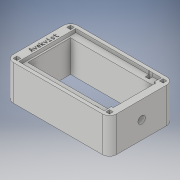
# Autodesk Inventor part: AttendMiddle
Saved by Autodesk Inventor 2019 (Build 230136000, 136)
## iProperties
Created: 2018-11-13
Part Number: AttendMiddle
Material: Generic
Document SubType Name: Modeling
Designer: hampu
Density: 1 g/cm^3
Appearance: Default
Author: hampu
Autodesk Inventor part; units mm, degrees
ref_plane "YZ Plane" through (0, 0, 0) normal (1, 0, 0) x (0, 1, 0)
ref_plane "XZ Plane" through (0, 0, 0) normal (0, 1, 0) x (-1, 0, 0)
ref_plane "XY Plane" through (0, 0, 0) normal (0, 0, 1) x (1, 0, 0)
sketch "Sketch1" plane through (0, 0, 0) normal (0, 1, 0) x (-1, 0, 0)
  line L0 (36.595, -22.775) -> (-36.595, -22.775)
  line L1 (-36.595, -22.775) -> (-36.595, 22.775)
  line L2 (-36.595, 22.775) -> (36.595, 22.775)
  line L3 (36.595, 22.775) -> (36.595, -22.775)
  line L4 (36.595, -22.775) -> (-36.595, 22.775) construction
  line L5 (-36.595, -22.775) -> (36.595, 22.775) construction
  line L6 (34.195, -17.675) -> (31.495, -17.675)
  line L7 (31.495, -17.675) -> (31.495, -20.375)
  line L8 (31.495, -20.375) -> (34.195, -20.375)
  line L9 (34.195, -20.375) -> (34.195, -17.675)
  line L10 (-24.195, -17.675) -> (-21.495, -17.675)
  line L11 (-21.495, -17.675) -> (-21.495, -20.375)
  line L12 (-21.495, -20.375) -> (-24.195, -20.375)
  line L13 (-24.195, -20.375) -> (-24.195, -17.675)
  line L14 (-21.495, 20.375) -> (-24.195, 20.375)
  line L15 (-24.195, 20.375) -> (-24.195, 17.675)
  line L16 (-24.195, 17.675) -> (-21.495, 17.675)
  line L17 (-21.495, 17.675) -> (-21.495, 20.375)
  line L18 (31.495, 20.375) -> (34.195, 20.375)
  line L19 (34.195, 20.375) -> (34.195, 17.675)
  line L20 (34.195, 17.675) -> (31.495, 17.675)
  line L21 (31.495, 17.675) -> (31.495, 20.375)
  line L22 (28.995, -15.175) -> (-18.995, -15.175)
  line L23 (-18.995, -15.175) -> (-18.995, 15.175)
  line L24 (-18.995, 15.175) -> (28.995, 15.175)
  line L25 (28.995, 15.175) -> (28.995, -15.175)
  line L26 (-18.995, 15.175) -> (-31.595, 15.175)
  line L27 (-31.595, 15.175) -> (-31.595, -15.175)
  line L28 (-31.595, -15.175) -> (-18.995, -15.175)
  line L29 (-18.995, -15.175) -> (-18.995, 15.175)
  point P0 (0, 0)
  dimension "d0" = 73.19
  dimension "d1" = 45.55
  dimension "d12" = 47.99
  dimension "d13" = 30.35
  dimension "d14" = 12.6
  constraints: 60 end point, 14 parallel, 7 perpendicular, 3 horizontal, 2 midpoint, 1 point on line
  measures "d0" distance of L1.end L2.end
  measures "d1" distance of L0.end L1.end
  measures "d12" distance of L23.end L24.end
  measures "d13" distance of L22.end L23.end
  measures "d14" distance of L28.end L27.end
extrude "Extrusion1" add sketch "Sketch1" along normal blind 25
sketch "Sketch4" plane through (0, 25, 0) normal (0, 1, 0) x (1, 0, 0)
  line L0 (-30, 20) -> (30, -20) construction
  line L1 (30, 20) -> (-30, -20) construction
  line L2 (30.3, 20.3) -> (-30.3, 20.3)
  line L3 (-30.3, 20.3) -> (-30.3, -20.3)
  line L4 (-30.3, -20.3) -> (30.3, -20.3)
  line L5 (30.3, -20.3) -> (30.3, 20.3)
  point P0 (0, 0)
  dimension "d21" = 60
  dimension "d22" = 40
  constraints: 12 end point, 2 midpoint, 2 parallel, 1 perpendicular
  measures "d21" distance of L0.end L1.end
  measures "d22" distance of L1.start L0.end
extrude "Extrusion2" cut sketch "Sketch4" against normal blind 2.5
sketch "Sketch5" plane through (0, 25, 0) normal (0, 1, 0) x (1, 0, 0)
  line L0 (34.195, -17.675) -> (31.495, -17.675)
  line L1 (31.495, -17.675) -> (31.495, -20.375)
  line L2 (31.495, -20.375) -> (34.195, -20.375)
  line L3 (34.195, -20.375) -> (34.195, -17.675)
  line L4 (34.195, 17.675) -> (31.495, 17.675)
  line L5 (31.495, 17.675) -> (31.495, 20.375)
  line L6 (31.495, 20.375) -> (34.195, 20.375)
  line L7 (34.195, 20.375) -> (34.195, 17.675)
  point P0 (0, 0)
  constraints: 16 end point, 4 parallel, 2 perpendicular
extrude "Extrusion3" cut sketch "Sketch5" against normal blind 10
sketch "Sketch6" plane through (0, 25, 0) normal (0, 1, 0) x (1, 0, 0)
  line L0 (-31.495, -17.675) -> (-34.195, -17.675) projected
  line L1 (-31.495, 20.375) -> (-31.495, 17.675) projected
  line L2 (-34.195, -17.675) -> (-31.495, -17.675)
  line L3 (-31.495, -17.675) -> (-31.495, 17.675)
  line L4 (-31.495, 17.675) -> (-34.195, 17.675)
  line L5 (-34.195, 17.675) -> (-34.195, -17.675)
  line L6 (-34.495, -8.4481) -> (-31.495, -7.5607)
  line L7 (-31.495, -7.5607) -> (-31.495, -7.9569)
  line L8 (-31.495, -7.9569) -> (-32.4642, -8.2421)
  line L9 (-32.4642, -8.2421) -> (-32.4642, -9.0845)
  line L10 (-32.4642, -9.0845) -> (-31.495, -9.3671)
  line L11 (-31.495, -9.3671) -> (-31.495, -9.7606)
  line L12 (-31.495, -9.7606) -> (-34.495, -8.8759)
  line L13 (-34.495, -8.8759) -> (-34.495, -8.4481)
  line L14 (-32.7652, -9.0053) -> (-32.7652, -8.3187)
  line L15 (-32.7652, -8.3187) -> (-34.0672, -8.6567)
  line L16 (-34.0672, -8.6567) -> (-32.7652, -9.0053)
  spline S0 degree 2 poles (-31.8753, -6.1796) (-32.3533, -6.0053) (-33.7027, -5.5326) knots 0 0 0 1 1 1
  line L17 (-33.7027, -5.5326) -> (-33.7027, -5.1259)
  line L18 (-33.7027, -5.1259) -> (-31.495, -5.9868)
  line L19 (-31.495, -5.9868) -> (-31.495, -6.3961)
  line L20 (-31.495, -6.3961) -> (-33.7027, -7.2491)
  line L21 (-33.7027, -7.2491) -> (-33.7027, -6.8266)
  line L22 (-33.7027, -6.8266) -> (-31.8753, -6.1796)
  spline S1 degree 2 poles (-31.598, -4.125) (-31.7538, -4.3574) (-32.274, -4.5819) (-32.929, -4.5819) (-33.4519, -4.3732) (-33.7714, -3.9613) (-33.7714, -3.713) knots 0 0 0 1 2 3 4 5 5 5
  spline S2 degree 2 poles (-33.7714, -3.713) (-33.7714, -3.2456) (-33.1323, -2.8125) (-32.6649, -2.8125) knots 0 0 0 1 2 2 2
  line L23 (-32.6649, -2.8125) -> (-32.5408, -2.8125)
  line L24 (-32.5408, -2.8125) -> (-32.5408, -4.2095)
  spline S3 degree 2 poles (-32.5408, -4.2095) (-32.2027, -4.1989) (-31.7274, -3.882) (-31.7274, -3.5651) knots 0 0 0 1 2 2 2
  spline S4 degree 2 poles (-31.7274, -3.5651) (-31.7459, -3.3539) (-31.9571, -2.9762) knots 0 0 0 1 1 1
  line L25 (-31.9571, -2.9762) -> (-31.7063, -2.8548)
  spline S5 degree 2 poles (-31.7063, -2.8548) (-31.4448, -3.1162) (-31.4448, -3.5704) knots 0 0 0 1 1 1
  spline S6 degree 2 poles (-31.4448, -3.5704) (-31.4448, -3.8952) (-31.598, -4.125) knots 0 0 0 1 1 1
  spline S7 degree 2 poles (-32.8101, -3.1611) (-33.4888, -3.2007) (-33.4888, -3.6364) knots 0 0 0 1 1 1
  spline S8 degree 2 poles (-33.4888, -3.6364) (-33.4888, -4.1276) (-32.8101, -4.1989) knots 0 0 0 1 1 1
  line L26 (-32.8101, -4.1989) -> (-32.8101, -3.1611)
  line L27 (-32.8075, -1.6849) -> (-33.7027, -0.7077)
  line L28 (-33.7027, -0.7077) -> (-33.7027, -0.243)
  line L29 (-33.7027, -0.243) -> (-32.7864, -1.228)
  line L30 (-32.7864, -1.228) -> (-31.495, -0.1083)
  line L31 (-31.495, -0.1083) -> (-31.495, -0.5678)
  line L32 (-31.495, -0.5678) -> (-32.6174, -1.4894)
  line L33 (-32.6174, -1.4894) -> (-32.4457, -1.6849)
  line L34 (-32.4457, -1.6849) -> (-31.495, -1.6849)
  line L35 (-31.495, -1.6849) -> (-31.495, -2.0519)
  line L36 (-31.495, -2.0519) -> (-34.6059, -2.0519)
  line L37 (-34.6059, -2.0519) -> (-34.6455, -1.6849)
  line L38 (-34.6455, -1.6849) -> (-32.8075, -1.6849)
  spline S9 degree 2 poles (-31.8753, 1.2438) (-32.3533, 1.4181) (-33.7027, 1.8908) knots 0 0 0 1 1 1
  line L39 (-33.7027, 1.8908) -> (-33.7027, 2.2975)
  line L40 (-33.7027, 2.2975) -> (-31.495, 1.4366)
  line L41 (-31.495, 1.4366) -> (-31.495, 1.0273)
  line L42 (-31.495, 1.0273) -> (-33.7027, 0.1743)
  line L43 (-33.7027, 0.1743) -> (-33.7027, 0.5968)
  line L44 (-33.7027, 0.5968) -> (-31.8753, 1.2438)
  line L45 (-33.4202, 2.9868) -> (-33.7027, 2.9868)
  line L46 (-33.7027, 2.9868) -> (-33.7027, 3.985)
  line L47 (-33.7027, 3.985) -> (-31.7776, 3.985)
  line L48 (-31.7776, 3.985) -> (-31.7776, 4.6162)
  line L49 (-31.7776, 4.6162) -> (-31.495, 4.6162)
  line L50 (-31.495, 4.6162) -> (-31.495, 2.9181)
  line L51 (-31.495, 2.9181) -> (-31.7776, 2.9181)
  line L52 (-31.7776, 2.9181) -> (-31.7776, 3.618)
  line L53 (-31.7776, 3.618) -> (-33.4202, 3.618)
  line L54 (-33.4202, 3.618) -> (-33.4202, 2.9868)
  line L55 (-34.2837, 3.5572) -> (-34.4844, 3.5572)
  spline S10 degree 2 poles (-34.4844, 3.5572) (-34.5557, 3.5572) (-34.6667, 3.721) (-34.6667, 3.882) (-34.5557, 4.0458) (-34.4844, 4.0458) knots 0 0 0 1 2 3 4 4 4
  line L56 (-34.4844, 4.0458) -> (-34.2837, 4.0458)
  spline S11 degree 2 poles (-34.2837, 4.0458) (-34.2124, 4.0458) (-34.1015, 3.882) (-34.1015, 3.721) (-34.2124, 3.5572) (-34.2837, 3.5572) knots 0 0 0 1 2 3 4 4 4
  spline S12 degree 2 poles (-32.7494, 6.4542) (-32.6781, 6.7394) (-32.3718, 7.0035) (-31.7961, 7.0035) (-31.4448, 6.5625) (-31.4448, 6.2324) knots 0 0 0 1 2 3 4 4 4
  spline S13 degree 2 poles (-31.4448, 6.2324) (-31.4448, 5.9947) (-31.5637, 5.5458) (-31.6429, 5.4401) knots 0 0 0 1 2 2 2
  line L57 (-31.6429, 5.4401) -> (-31.907, 5.5299)
  spline S14 degree 2 poles (-31.907, 5.5299) (-31.8542, 5.6144) (-31.7485, 5.9815) (-31.7485, 6.4093) (-31.9281, 6.6655) (-32.2265, 6.6655) (-32.3955, 6.5387) (-32.4404, 6.3592) knots 0 0 0 1 2 3 4 5 6 6 6
  line L58 (-32.4404, 6.3592) -> (-32.5329, 5.9842)
  spline S15 degree 2 poles (-32.5329, 5.9842) (-32.6121, 5.6593) (-32.9211, 5.4454) (-33.3779, 5.4454) (-33.7661, 5.8178) (-33.7688, 6.1743) knots 0 0 0 1 2 3 4 4 4
  line L59 (-33.7688, 6.1743) -> (-33.7688, 6.2007)
  spline S16 degree 2 poles (-33.7688, 6.2007) (-33.7688, 6.6021) (-33.6182, 6.882) knots 0 0 0 1 1 1
  line L60 (-33.6182, 6.882) -> (-33.3621, 6.8028)
  spline S17 degree 2 poles (-33.3621, 6.8028) (-33.4862, 6.5097) (-33.4862, 6.206) knots 0 0 0 1 1 1
  spline S18 degree 2 poles (-33.4862, 6.206) (-33.4836, 6.0211) (-33.3013, 5.7808) (-33.024, 5.7808) (-32.8841, 5.9023) (-32.8445, 6.0713) knots 0 0 0 1 2 3 4 4 4
  line L61 (-32.8445, 6.0713) -> (-32.7494, 6.4542)
  line L62 (-33.4202, 8.596) -> (-32.385, 8.596)
  spline S19 degree 2 poles (-32.385, 8.596) (-32.1922, 8.596) (-31.9651, 8.6382) (-31.8251, 8.765) (-31.7776, 8.9683) (-31.7776, 9.14) knots 0 0 0 1 2 3 4 4 4
  line L63 (-31.7776, 9.14) -> (-31.7776, 9.544)
  line L64 (-31.7776, 9.544) -> (-31.495, 9.5255)
  line L65 (-31.495, 9.5255) -> (-31.495, 9.1558)
  spline S20 degree 2 poles (-31.495, 9.1558) (-31.495, 8.5854) (-31.7036, 8.3952) knots 0 0 0 1 1 1
  spline S21 degree 2 poles (-31.7036, 8.3952) (-31.841, 8.2738) (-32.1446, 8.2447) knots 0 0 0 1 1 1
  spline S22 degree 2 poles (-32.1446, 8.2447) (-32.2793, 8.2315) (-32.4774, 8.2315) knots 0 0 0 1 1 1
  line L66 (-32.4774, 8.2315) -> (-33.4202, 8.2315)
  line L67 (-33.4202, 8.2315) -> (-33.4202, 7.6056)
  line L68 (-33.4202, 7.6056) -> (-33.7027, 7.6479)
  line L69 (-33.7027, 7.6479) -> (-33.7027, 8.2315)
  line L70 (-33.7027, 8.2315) -> (-34.4633, 8.2315)
  line L71 (-34.4633, 8.2315) -> (-34.5716, 8.596)
  line L72 (-34.5716, 8.596) -> (-33.7027, 8.596)
  line L73 (-33.7027, 8.596) -> (-33.7027, 9.5282)
  line L74 (-33.7027, 9.5282) -> (-33.4202, 9.5282)
  line L75 (-33.4202, 9.5282) -> (-33.4202, 8.596)
  point P0 (0, 0)
  constraints: 8 end point, 2 parallel, 1 horizontal, 1 perpendicular, 1 vertical
extrude "Extrusion4" cut sketch "Sketch6" against normal blind 2 contours L12 L5 L6 L3 L8 L9 L10 | L12 L13 L6 L5 | L36 L37 L38 L5 | L5 L38 L27 L28 L29 L30 L3 L32 L33 L34 L36 | L20 L21 L22 S0 L17 L18 L3 | S11 L55 S10 L56 L5 | L5 S11 | S5 S6 L3 | L3 S6 S1 S2 L23 L24 S3 S4 L25 S5 | L70 L71 L72 L5 | L5 L72 L73 L74 L75 L62 S19 L63 L64 L3 S20 S21 S22 L66 L67 L68 L69 L70 | L42 L43 L44 S9 L39 L40 L3 | L51 L52 L53 L54 L45 L46 L47 L48 L49 L3 | S13 L57 S14 L58 S15 L59 S16 L60 S17 S18 L61 S12 L3 | L3 S12 S13
fillet "Fillet1" radius 5 4 edges at (36.595, 12.5, -22.775) (36.595, 12.5, 22.775) (-36.595, 12.5, -22.775) (-36.595, 12.5, 22.775)
sketch "Sketch7" plane through (36.595, 0, 17.775) normal (1, 0, 0) x (0, 0, -1)
  line L0 (12.775, 17.5) -> (22.775, 17.5)
  line L1 (22.775, 17.5) -> (22.775, 7.5)
  line L2 (22.775, 7.5) -> (12.775, 7.5)
  line L3 (12.775, 7.5) -> (12.775, 17.5)
  line L4 (12.775, 17.5) -> (22.775, 7.5) construction
  line L5 (22.775, 17.5) -> (12.775, 7.5) construction
  circle A0 centre (17.775, 12.5) radius 2.6
  point P0 (17.775, 0)
  dimension "d37" = 10
  dimension "d38" = 10
  dimension "d39" = 5.2
  constraints: 12 end point, 2 midpoint, 2 parallel, 1 centre point, 1 coincident, 1 horizontal, 1 perpendicular
  measures "d37" distance of L1.end L2.end
  measures "d38" distance of L0.end L1.end
  measures "d39" diameter of A0
extrude "Extrusion5" cut sketch "Sketch7" against normal blind 5 contours A0
body "Solid1"
